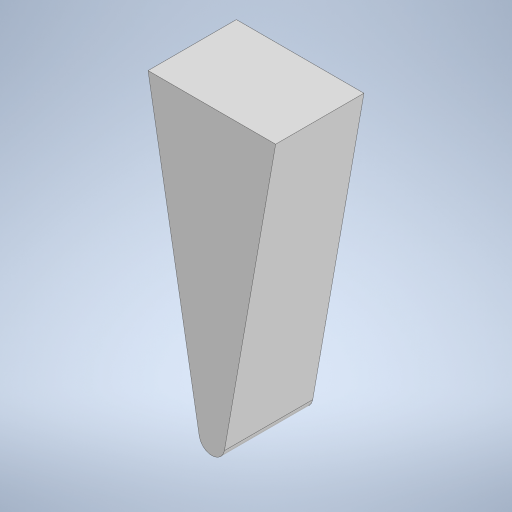
# Autodesk Inventor part: finley_gripper_60
Saved by Autodesk Inventor 2024 (Build 280153000, 153)
## iProperties
Created: 2024-09-23
Part Number: finley_gripper_60
Material: 一般
Document SubType Name: Modeling
Designer: 1412z
Density: 1 g/cm^3
Appearance: 既定
Author: 1412z
Autodesk Inventor part; units mm, degrees
ref_plane "YZ Plane" through (0, 0, 0) normal (1, 0, 0) x (0, 1, 0)
ref_plane "XZ Plane" through (0, 0, 0) normal (0, 1, 0) x (-1, 0, 0)
ref_plane "XY Plane" through (0, 0, 0) normal (0, 0, 1) x (1, 0, 0)
sketch "スケッチ1" plane through (0, 0, 0) normal (0, 0, 1) x (1, 0, 0)
  line L0 (0, 0) -> (-26, 0)
  line L1 (0, 0) -> (-13, -73.8647)
  line L2 (-13, -73.8647) -> (-26, 0)
  dimension "d0" = 26
  dimension "d1" = 75
  constraints: 6 end point, 1 horizontal
  measures "d0" distance of L0.start L0.end
  measures "d1" distance of L0.start L1.end
extrude "押し出し1" add sketch "スケッチ1" along normal mid plane 18
fillet "フィレット1" radius 2.6 1 edges at (-13, -73.8647, 0)
